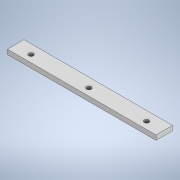
# Autodesk Inventor part: Seal
Saved by Autodesk Inventor 2020.1 (Build 241239000, 239)
## iProperties
Created: 2022-02-14
Part Number: Seal
Material: Generic
Document SubType Name: Modeling
Designer: OEM
Density: 1 g/cm^3
Appearance: Default
Author: OEM
Autodesk Inventor part; units mm, degrees
ref_plane "YZ Plane" through (0, 0, 0) normal (1, 0, 0) x (0, 1, 0)
ref_plane "XZ Plane" through (0, 0, 0) normal (0, 1, 0) x (-1, 0, 0)
ref_plane "XY Plane" through (0, 0, 0) normal (0, 0, 1) x (1, 0, 0)
sketch "Sketch1" plane through (0, 0, 0) normal (0, 1, 0) x (-1, 0, 0)
  line L0 (0, 0) -> (63, 0)
  line L1 (63, 0) -> (63, -7)
  line L2 (63, -7) -> (0, -7)
  line L3 (0, -7) -> (0, 0)
  circle A0 centre (31.5, -3) radius 1
  line L4 (31.5, 0) -> (31.5, -6) construction
  circle A1 centre (7, -3) radius 1
  circle A2 centre (56, -3) radius 1
  line L5 (63, -3) -> (0, -3) construction
  dimension "d0" = 63
  dimension "d1" = 7
  dimension "d2" = 2
  dimension "d3" = 31.5
  dimension "d5" = 7
  dimension "d6" = 2
  dimension "d9" = 3
  constraints: 12 end point, 3 centre point, 3 perpendicular, 2 parallel, 2 point on line, 1 horizontal, 1 midpoint, 1 symmetric about line, 1 other
  measures "d0" distance of L1.end L2.end
  measures "d1" distance of L0.end L1.end
  measures "d2" diameter of A0
  measures "d3" distance from line of A0.centre L3
  measures "d5" distance from line of A1.centre L3
  measures "d6" diameter of A1
  measures "d9" distance from line of L0 A2.centre
extrude "Extrusion1" add sketch "Sketch1" along normal blind 2
equation "\"d3\" = 0.5 * d0"
equation "\"d6\" = d2"
body "Solid1"
